Autodesk Inventor part; units mm, degrees
(part 2 of 2)
revolve "Revolution35" add sketch "Sketch_83" angle 360 about axis through (298.5, 17.5, 82.5) along (-1, 0, 0)
thread "Thread5" size "M8x1.25" class "6g" standard "ISO Metric profile" length 12.983
sketch "Sketch_108" plane through (0, 0, 159.75) normal (0, 0, 1) x (1, 0, 0)
  line L0 (282.4, 697.5) -> (276.2, 697.5)
  line L1 (276.2, 697.5) -> (276.2, 702)
  line L2 (276.2, 702) -> (278, 702)
  line L3 (278, 702) -> (278, 700.5)
  line L4 (278, 700.5) -> (278.7, 700.5)
  line L5 (278.7, 700.5) -> (278.7, 700)
  line L6 (278.7, 700) -> (281.9095, 700)
  line L7 (281.9095, 700) -> (282.4, 699.5095)
  line L8 (282.4, 699.5095) -> (282.4, 697.5)
  line L9 (282.4, 697.5) -> (276.2, 697.5)
  constraints: 20 end point
revolve "Revolution36" add sketch "Sketch_108" angle 360 about axis through (282.4, 697.5, 159.75) along (1, 0, 0)
thread "Thread6" size "M5x0.8" class "6g" standard "ISO Metric profile" full length
sketch "Sketch_109" plane through (0, 0, 159.75) normal (0, 0, 1) x (1, 0, 0)
  line L0 (282.4, 62.5) -> (276.2, 62.5)
  line L1 (276.2, 62.5) -> (276.2, 67)
  line L2 (276.2, 67) -> (278, 67)
  line L3 (278, 67) -> (278, 65.5)
  line L4 (278, 65.5) -> (278.7, 65.5)
  line L5 (278.7, 65.5) -> (278.7, 65)
  line L6 (278.7, 65) -> (281.9095, 65)
  line L7 (281.9095, 65) -> (282.4, 64.5095)
  line L8 (282.4, 64.5095) -> (282.4, 62.5)
  line L9 (282.4, 62.5) -> (276.2, 62.5)
  constraints: 20 end point
revolve "Revolution37" add sketch "Sketch_109" angle 360 about axis through (282.4, 62.5, 159.75) along (1, 0, 0)
thread "Thread7" size "M5x0.8" class "6g" standard "ISO Metric profile" full length
sketch "Sketch73" plane through (297, 3, -175) normal (0, 0, -1) x (-1, 0, 0)
  point P0 (7, 59.5)
hole "Hole5" at (290, 62.5, -175) direction (0, 0, 1) diameter 10 depth 1.5
pattern_linear "Rectangular Pattern1" count 3 spacing 317.5 along (0, 1, 0) count 2 spacing 580 along (-1, 0, 0) of "Hole5"
sketch "Sketch74" plane through (297, 3, -175) normal (0, 0, -1) x (-1, 0, 0)
  point P0 (59.5, 7)
hole "Hole6" at (237.5, 10, -175) direction (0, 0, 1) diameter 10 depth 1.5
pattern_linear "Rectangular Pattern2" count 2 spacing 740 along (0, 1, 0) count 3 spacing 237.5 along (-1, 0, 0) of "Hole6"
sketch "Sketch75" plane through (-297, 757, 152.5) normal (0, 0, 1) x (1, 0, 0)
  point P0 (587, -694.5)
hole "Hole7" at (290, 62.5, 152.5) direction (0, 0, -1) diameter 10 depth 1.5
pattern_linear "Rectangular Pattern3" count 3 spacing 317.5 along (0, 1, 0) count 2 spacing 580 along (-1, 0, 0) of "Hole7"
sketch "Sketch76" plane through (-297, 757, 152.5) normal (0, 0, 1) x (1, 0, 0)
  point P0 (534.5, -747)
hole "Hole8" at (237.5, 10, 152.5) direction (0, 0, -1) diameter 10 depth 1.5
pattern_linear "Rectangular Pattern4" count 2 spacing 740 along (0, 1, 0) count 3 spacing 237.5 along (-1, 0, 0) of "Hole8"
sketch "Sketch_128" plane through (0, 10, 0) normal (0, 1, 0) x (1, 0, 0)
  line L0 (237.5, 171.7) -> (237.5, 175)
  line L1 (237.5, 173.2) -> (239.902, 173.2)
  arc A0 (239.902, 173.2) -> (240.3995, 173.65) centre (239.902, 173.7) ccw
  arc A1 (241.892, 175) -> (240.3995, 173.65) centre (241.892, 173.5) ccw
  line L2 (241.892, 175) -> (243.5, 175)
  line L3 (243.5, 175) -> (243.5, 173.5)
  line L4 (243.5, 173.5) -> (241.6685, 173.5)
  arc A2 (241.6685, 173.5) -> (240.7741, 172.9472) centre (241.6685, 172.5) ccw
  line L5 (240.7741, 172.9472) -> (240.551, 172.501)
  arc A3 (239.571, 171.7) -> (240.551, 172.501) centre (239.571, 172.7) ccw
  line L6 (239.571, 171.7) -> (237.5, 171.7)
  line L7 (237.5, 171.7) -> (237.5, 173.2)
  constraints: 16 end point, 8 point on circle, 4 centre point
revolve "Revolution38" add sketch "Sketch_128" angle 360 about axis through (237.5, 10, -171.7) along (0, 0, 1)
pattern_linear "Rectangular Pattern5" count 2 spacing 740 along (0, 1, 0) count 3 spacing 237.5 along (-1, 0, 0) of "Revolution38"
sketch "Sketch_130" plane through (0, 62.5, 0) normal (0, 1, 0) x (1, 0, 0)
  line L0 (290, 171.7) -> (290, 175)
  line L1 (290, 173.2) -> (292.402, 173.2)
  arc A0 (292.402, 173.2) -> (292.8995, 173.65) centre (292.402, 173.7) ccw
  arc A1 (294.392, 175) -> (292.8995, 173.65) centre (294.392, 173.5) ccw
  line L2 (294.392, 175) -> (296, 175)
  line L3 (296, 175) -> (296, 173.5)
  line L4 (296, 173.5) -> (294.1685, 173.5)
  arc A2 (294.1685, 173.5) -> (293.2741, 172.9472) centre (294.1685, 172.5) ccw
  line L5 (293.2741, 172.9472) -> (293.051, 172.501)
  arc A3 (292.071, 171.7) -> (293.051, 172.501) centre (292.071, 172.7) ccw
  line L6 (292.071, 171.7) -> (290, 171.7)
  line L7 (290, 171.7) -> (290, 173.2)
  constraints: 16 end point, 8 point on circle, 4 centre point
revolve "Revolution39" add sketch "Sketch_130" angle 360 about axis through (290, 62.5, -171.7) along (0, 0, 1)
pattern_linear "Rectangular Pattern6" count 3 spacing 317.5 along (0, 1, 0) count 2 spacing 580 along (-1, 0, 0) of "Revolution39"
sketch "Sketch_132" plane through (0, 10, 0) normal (0, 1, 0) x (1, 0, 0)
  line L0 (237.5, -152.5) -> (237.5, -149.2)
  line L1 (237.5, -149.2) -> (239.571, -149.2)
  arc A0 (240.551, -150.001) -> (239.571, -149.2) centre (239.571, -150.2) ccw
  line L2 (240.551, -150.001) -> (240.7741, -150.4472)
  arc A1 (240.7741, -150.4472) -> (241.6685, -151) centre (241.6685, -150) ccw
  line L3 (241.6685, -151) -> (243.5, -151)
  line L4 (243.5, -151) -> (243.5, -152.5)
  line L5 (243.5, -152.5) -> (241.892, -152.5)
  arc A2 (240.3995, -151.15) -> (241.892, -152.5) centre (241.892, -151) ccw
  arc A3 (240.3995, -151.15) -> (239.902, -150.7) centre (239.902, -151.2) ccw
  line L6 (239.902, -150.7) -> (237.5, -150.7)
  line L7 (237.5, -150.7) -> (237.5, -149.2)
  constraints: 16 end point, 8 point on circle, 4 centre point
revolve "Revolution40" add sketch "Sketch_132" angle 360 about axis through (237.5, 10, 152.5) along (0, 0, 1)
pattern_linear "Rectangular Pattern7" count 2 spacing 740 along (0, 1, 0) count 3 spacing 237.5 along (-1, 0, 0) of "Revolution40"
sketch "Sketch_134" plane through (0, 62.5, 0) normal (0, 1, 0) x (1, 0, 0)
  line L0 (290, -152.5) -> (290, -149.2)
  line L1 (290, -149.2) -> (292.071, -149.2)
  arc A0 (293.051, -150.001) -> (292.071, -149.2) centre (292.071, -150.2) ccw
  line L2 (293.051, -150.001) -> (293.2741, -150.4472)
  arc A1 (293.2741, -150.4472) -> (294.1685, -151) centre (294.1685, -150) ccw
  line L3 (294.1685, -151) -> (296, -151)
  line L4 (296, -151) -> (296, -152.5)
  line L5 (296, -152.5) -> (294.392, -152.5)
  arc A2 (292.8995, -151.15) -> (294.392, -152.5) centre (294.392, -151) ccw
  arc A3 (292.8995, -151.15) -> (292.402, -150.7) centre (292.402, -151.2) ccw
  line L6 (292.402, -150.7) -> (290, -150.7)
  line L7 (290, -150.7) -> (290, -149.2)
  constraints: 16 end point, 8 point on circle, 4 centre point
revolve "Revolution41" add sketch "Sketch_134" angle 360 about axis through (290, 62.5, 152.5) along (0, 0, 1)
pattern_linear "Rectangular Pattern8" count 3 spacing 317.5 along (0, 1, 0) count 2 spacing 580 along (-1, 0, 0) of "Revolution41"
ref_plane "FP1_XY" through (0, -0.5, -45.5) normal (0, 1, 0) x (1, 0, 0)
ref_plane "FP1_YZ" through (0, -0.5, -45.5) normal (1, 0, 0) x (0, 0, -1)
ref_plane "FP1_ZX" through (0, -0.5, -45.5) normal (0, 0, -1) x (0, 1, 0)
ref_plane "FP2_XY" through (0, -0.5, -45.5) normal (0, 1, 0) x (1, 0, 0)
ref_plane "FP2_YZ" through (0, -0.5, -45.5) normal (1, 0, 0) x (0, 0, -1)
ref_plane "FP2_ZX" through (0, -0.5, -45.5) normal (0, 0, -1) x (0, 1, 0)
ref_plane "GEHAEUSE_XY" through (0, 380, -175) normal (0, 1, 0) x (1, 0, 0)
ref_plane "GEHAEUSE_YZ" through (0, 380, -175) normal (1, 0, 0) x (0, 0, -1)
ref_plane "GEHAEUSE_ZX" through (0, 380, -175) normal (0, 0, -1) x (0, 1, 0)
ref_plane "MP_XY" through (0, 25, -155) normal (0, 0, -1) x (1, 0, 0)
ref_plane "MP_YZ" through (0, 25, -155) normal (1, 0, 0) x (0, -1, 0)
ref_plane "MP_ZX" through (0, 25, -155) normal (0, -1, 0) x (0, 0, -1)
ref_plane "REVIT_XY" through (0, 0, -175) normal (0, 0, -1) x (1, 0, 0)
ref_plane "REVIT_YZ" through (0, 0, -175) normal (1, 0, 0) x (0, -1, 0)
ref_plane "REVIT_ZX" through (0, 0, -175) normal (0, -1, 0) x (0, 0, -1)
ref_plane "SCLM_XY" through (-279.5, 380, 159.75) normal (1, 0, 0) x (0, 0, -1)
ref_plane "SCLM_YZ" through (-279.5, 380, 159.75) normal (0, 0, -1) x (0, 1, 0)
ref_plane "SCLM_ZX" through (-279.5, 380, 159.75) normal (0, 1, 0) x (1, 0, 0)
ref_plane "SCLO_XY" through (-279.5, 697.5, 159.75) normal (1, 0, 0) x (0, 0, -1)
ref_plane "SCLO_YZ" through (-279.5, 697.5, 159.75) normal (0, 0, -1) x (0, 1, 0)
ref_plane "SCLO_ZX" through (-279.5, 697.5, 159.75) normal (0, 1, 0) x (1, 0, 0)
ref_plane "SCLU_XY" through (-279.5, 62.5, 159.75) normal (1, 0, 0) x (0, 0, -1)
ref_plane "SCLU_YZ" through (-279.5, 62.5, 159.75) normal (0, 0, -1) x (0, 1, 0)
ref_plane "SCLU_ZX" through (-279.5, 62.5, 159.75) normal (0, 1, 0) x (1, 0, 0)
ref_plane "SCRM_XY" through (279.5, 380, 159.75) normal (-1, 0, 0) x (0, 0, -1)
ref_plane "SCRM_YZ" through (279.5, 380, 159.75) normal (0, 0, -1) x (0, -1, 0)
ref_plane "SCRM_ZX" through (279.5, 380, 159.75) normal (0, -1, 0) x (-1, 0, 0)
ref_plane "SCRO_XY" through (279.5, 697.5, 159.75) normal (-1, 0, 0) x (0, 0, -1)
ref_plane "SCRO_YZ" through (279.5, 697.5, 159.75) normal (0, 0, -1) x (0, -1, 0)
ref_plane "SCRO_ZX" through (279.5, 697.5, 159.75) normal (0, -1, 0) x (-1, 0, 0)
ref_plane "SCRU_XY" through (279.5, 62.5, 159.75) normal (-1, 0, 0) x (0, 0, -1)
ref_plane "SCRU_YZ" through (279.5, 62.5, 159.75) normal (0, 0, -1) x (0, -1, 0)
ref_plane "SCRU_ZX" through (279.5, 62.5, 159.75) normal (0, -1, 0) x (-1, 0, 0)
ref_plane "to_Abst_tzung_L_XY" through (-250, 25, -146.75) normal (0, 0, 1) x (1, 0, 0)
ref_plane "to_Abst_tzung_L_YZ" through (-250, 25, -146.75) normal (1, 0, 0) x (0, 1, 0)
ref_plane "to_Abst_tzung_L_ZX" through (-250, 25, -146.75) normal (0, 1, 0) x (0, 0, 1)
ref_plane "to_Abst_tzung_R_XY" through (250, 25, -146.75) normal (0, 0, 1) x (1, 0, 0)
ref_plane "to_Abst_tzung_R_YZ" through (250, 25, -146.75) normal (1, 0, 0) x (0, 1, 0)
ref_plane "to_Abst_tzung_R_ZX" through (250, 25, -146.75) normal (0, 1, 0) x (0, 0, 1)
ref_plane "to_Cap_1_XY" through (280, 20, -175) normal (0, 0, 1) x (1, 0, 0)
ref_plane "to_Cap_1_YZ" through (280, 20, -175) normal (1, 0, 0) x (0, 1, 0)
ref_plane "to_Cap_1_ZX" through (280, 20, -175) normal (0, 1, 0) x (0, 0, 1)
ref_plane "to_Cap_2_XY" through (-280, 20, -175) normal (0, 0, 1) x (1, 0, 0)
ref_plane "to_Cap_2_YZ" through (-280, 20, -175) normal (1, 0, 0) x (0, 1, 0)
ref_plane "to_Cap_2_ZX" through (-280, 20, -175) normal (0, 1, 0) x (0, 0, 1)
ref_plane "to_Cap_3_XY" through (280, 740, -175) normal (0, 0, 1) x (1, 0, 0)
ref_plane "to_Cap_3_YZ" through (280, 740, -175) normal (1, 0, 0) x (0, 1, 0)
ref_plane "to_Cap_3_ZX" through (280, 740, -175) normal (0, 1, 0) x (0, 0, 1)
ref_plane "to_Cap_4_XY" through (-280, 740, -175) normal (0, 0, 1) x (1, 0, 0)
ref_plane "to_Cap_4_YZ" through (-280, 740, -175) normal (1, 0, 0) x (0, 1, 0)
ref_plane "to_Cap_4_ZX" through (-280, 740, -175) normal (0, 1, 0) x (0, 0, 1)
ref_plane "to_Plug_XY" through (-283.5, 0, 136) normal (0, 1, 0) x (1, 0, 0)
ref_plane "to_Plug_YZ" through (-283.5, 0, 136) normal (1, 0, 0) x (0, 0, -1)
ref_plane "to_Plug_ZX" through (-283.5, 0, 136) normal (0, 0, -1) x (0, 1, 0)
ref_plane "to_Plug_3_XY" through (250, 760, -53.5) normal (0, 1, 0) x (1, 0, 0)
ref_plane "to_Plug_3_YZ" through (250, 760, -53.5) normal (1, 0, 0) x (0, 0, -1)
ref_plane "to_Plug_3_ZX" through (250, 760, -53.5) normal (0, 0, -1) x (0, 1, 0)
ref_plane "to_Plug_4_XY" through (-250, 760, -53.5) normal (0, 1, 0) x (1, 0, 0)
ref_plane "to_Plug_4_YZ" through (-250, 760, -53.5) normal (1, 0, 0) x (0, 0, -1)
ref_plane "to_Plug_4_ZX" through (-250, 760, -53.5) normal (0, 0, -1) x (0, 1, 0)
ref_plane "to_Plug_1_1_XY" through (255, 0, -130) normal (0, 1, 0) x (1, 0, 0)
ref_plane "to_Plug_1_1_YZ" through (255, 0, -130) normal (1, 0, 0) x (0, 0, -1)
ref_plane "to_Plug_1_1_ZX" through (255, 0, -130) normal (0, 0, -1) x (0, 1, 0)
ref_plane "to_Plug_1_2_XY" through (-255, 0, -130) normal (0, 1, 0) x (1, 0, 0)
ref_plane "to_Plug_1_2_YZ" through (-255, 0, -130) normal (1, 0, 0) x (0, 0, -1)
ref_plane "to_Plug_1_2_ZX" through (-255, 0, -130) normal (0, 0, -1) x (0, 1, 0)
ref_plane "to_Plug_1_3_XY" through (255, 0, 57.5) normal (0, 1, 0) x (1, 0, 0)
ref_plane "to_Plug_1_3_YZ" through (255, 0, 57.5) normal (1, 0, 0) x (0, 0, -1)
ref_plane "to_Plug_1_3_ZX" through (255, 0, 57.5) normal (0, 0, -1) x (0, 1, 0)
ref_plane "to_Plug_1_4_XY" through (-255, 0, 57.5) normal (0, 1, 0) x (1, 0, 0)
ref_plane "to_Plug_1_4_YZ" through (-255, 0, 57.5) normal (1, 0, 0) x (0, 0, -1)
ref_plane "to_Plug_1_4_ZX" through (-255, 0, 57.5) normal (0, 0, -1) x (0, 1, 0)
body "Solid1"
